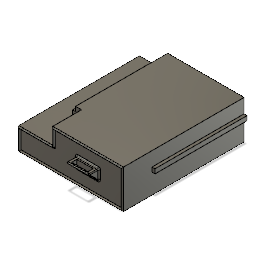
Drawer_for_ender3-pro_v14 (Autodesk Fusion 360 design; units mm, degrees)
Autodesk Fusion 360 part; units mm, degrees
sketch "Sketch1" plane through (0, 0, 0) normal (0, 0, 1) x (1, 0, 0)
  line L0 (0, 0) -> (-103, 0)
  line L1 (-103, 0) -> (-103, 52)
  line L2 (-103, 52) -> (0, 52)
  line L3 (0, 52) -> (0, 0)
  line L4 (0, 32.9) -> (4, 32.9)
  line L5 (4, 32.9) -> (4, 26.9)
  line L6 (4, 26.9) -> (0, 26.9)
  line L7 (-103, 46) -> (-107, 46)
  line L8 (-107, 46) -> (-107, 40)
  line L9 (-107, 40) -> (-103, 40)
  line L10 (-103, 30) -> (-141, 30)
  line L11 (-141, 30) -> (-141, 0)
  line L12 (-141, 0) -> (-103, 0)
  line L13 (-95, 52) -> (-95, 30)
  line L14 (-95, 30) -> (-103, 30)
  point P0 (0, 26.9)
  point P1 (0, 32.9)
  point P2 (-103, 40)
  point P3 (-103, 46)
  point P4 (-103, 30)
  point P5 (-95, 52)
  dimension "d1" = 103
  dimension "d2" = 52
  dimension "d3" = 26.9
  dimension "d4" = 6
  dimension "d5" = 4
  dimension "d6" = 40
  dimension "d7" = 6
  dimension "d8" = 4
  dimension "d9" = 30
  dimension "d10" = 38
  dimension "d11" = 8
  constraint horizontal L0
  constraint vertical L1
  constraint horizontal L2
  constraint vertical L3
  constraint coincident L0.start L3.end
  constraint coincident L3 P0
  constraint coincident L3 P1
  constraint coincident P1 L4.start
  constraint perpendicular L3 L4
  constraint perpendicular L4 L5
  constraint coincident P0 L6.end
  constraint perpendicular L3 L6
  constraint coincident L1 P2
  constraint coincident L1 P3
  constraint coincident P3 L7.start
  constraint horizontal L7
  constraint perpendicular L7 L8
  constraint coincident P2 L9.end
  constraint perpendicular L8 L9
  constraint coincident L1 P4
  constraint coincident P4 L10.start
  constraint perpendicular L1 L10
  constraint perpendicular L0 L11
  constraint perpendicular L1 L12
  constraint coincident L2 P5
  constraint coincident P5 L13.start
  constraint perpendicular L10 L13
  constraint perpendicular L1 L14
  measures "d1" distance of L0.start L0.end
  measures "d2" distance of L0.end L1.end
  measures "d3" distance of L0.start L6.end
  measures "d4" distance of P0 P1
  measures "d5" distance of P1 L4.end
  measures "d6" distance of L0.end L9.end
  measures "d7" distance of P2 P3
  measures "d8" distance of P3 L7.end
  measures "d9" distance of L0.end P4
  measures "d10" distance of P4 L10.end
  measures "d11" distance of L1.end P5
extrude "Extrude1" add sketch "Sketch1" along normal blind 164 contours L0 L1 L2 L3 L13 L14 | L1 L10 L11 L12 makes body 1
shell "Shell1" thickness 1.6 removed faces 1 at (-66, 10, 164) on bodies 1
extrude "Extrude2" add sketch "Sketch1" along normal blind 124 contours L3 L4 L5 L6 bodies 1
extrude "Extrude3" add sketch "Sketch1" along normal blind 124 contours L1 L2 L13 L14 | L1 L7 L8 L9 bodies 1
sketch "Sketch2" plane through (0, 0, 0) normal (0, 0, 1) x (1, 0, 0)
  line L0 (-95, 30) -> (-103, 30)
  line L1 (-95, 52) -> (-95, 30)
  line L2 (-95, 30) -> (-141, 30)
  line L3 (-141, 30) -> (-141, 0)
  line L4 (-141, 0) -> (0, 0)
  line L5 (0, 0) -> (0, 52)
  line L6 (0, 52) -> (-95, 52)
  line L7 (-93, 28) -> (-139, 28)
  line L8 (-139, 28) -> (-139, 2)
  line L9 (-139, 2) -> (-2, 2)
  line L10 (-2, 2) -> (-2, 50)
  line L11 (-2, 50) -> (-93, 50)
  line L12 (-93, 50) -> (-93, 28)
  point P0 (-95, 52)
  point P1 (-95, 30)
  point P2 (-141, 30)
  point P3 (-141, 0)
  point P4 (0, 52)
  dimension "d19" = 2
  constraint coincident P0 L1.start
  constraint coincident P1 L0.start
  constraint coincident P2 L2.end
  constraint coincident P3 L3.end
  constraint coincident L4.end L5.start
  constraint coincident P4 L5.end
extrude "Extrude4" add sketch "Sketch2" along normal blind 162.2 separate body contours L7 L8 L9 L10 L11 L12 makes body 2
shell "Shell2" thickness 1.6 removed faces 3 at (-32.3333, 50, 54.0667) at (-108.3333, 28, 108.1333) at (-93, 42.6667, 54.0667) on bodies 2
fillet "Fillet1" radius 1 10 edges at (-70.5, 2, 0) (-139, 15, 0) (-116, 28, 0) (-2, 26, 0) (-47.5, 50, 0) (-93, 39, 0) (-139, 28, 81.1) (-139, 2, 81.1) (-2, 2, 81.1) (-2, 50, 81.1) on bodies 2
fillet "Fillet2" radius 3 2 edges at (-93, 50, 1.3) (-92.7071, 49.7071, 0.2929) on bodies 2
fillet "Fillet3" radius 1 10 edges at (-115.5, 28, 162.2) (-138.7071, 27.7071, 162.2) (-139, 15, 162.2) (-138.7071, 2.2929, 162.2) (-70.5, 2, 162.2) (-2.2929, 2.2929, 162.2) (-2, 26, 162.2) (-2.2929, 49.7071, 162.2) (-48, 50, 162.2) (-93, 39, 162.2) on bodies 2
sketch "Sketch3" plane through (0, 0, 162.2) normal (0, 0, 1) x (1, 0, 0)
  line L0 (-3, 3) -> (-3, 49)
  line L1 (-3, 49) -> (-92, 49)
  line L2 (-92, 49) -> (-92, 27)
  line L3 (-92, 27) -> (-138, 27)
  line L4 (-138, 27) -> (-138, 3)
  line L5 (-138, 3) -> (-3, 3)
  line L6 (-33, 18.5) -> (-63, 18.5)
  line L7 (-63, 18.5) -> (-63, 33.5)
  line L8 (-63, 33.5) -> (-33, 33.5)
  line L9 (-33, 33.5) -> (-33, 18.5)
  line L10 (-33, 18.5) -> (-63, 33.5) construction
  line L11 (-63, 18.5) -> (-33, 33.5) construction
  point P0 (-48, 26)
  point P1 (-48, 26)
  point P2 (-48, 26)
  dimension "d34" = 30
  dimension "d35" = 15
  constraint coincident P2 P1
  constraint perpendicular L6 L7
  constraint parallel L6 L8
  constraint parallel L7 L9
  constraint horizontal L6
  constraint coincident L10 P2
  constraint coincident L11 P2
  measures "d34" distance of L7.end L8.end
  measures "d35" distance of L6.end L7.end
extrude "Extrude7" add sketch "Sketch3" along normal blind 15 contours L6 L7 L8 L9 bodies 2
sketch "Sketch5" plane through (-63, 0, 0) normal (-1, 0, 0) x (0, 0, 1)
  line L0 (162.2, 33.5) -> (162.2, 18.5)
  line L1 (162.2, 18.5) -> (177.2, 18.5)
  line L2 (177.2, 18.5) -> (177.2, 33.5)
  line L3 (177.2, 33.5) -> (162.2, 33.5)
  line L4 (162.2, 18.5) -> (177.2, 33.5)
  constraint coincident L0.end L1.start
  constraint coincident L2.end L3.start
extrude "Extrude8" cut sketch "Sketch5" against normal up to surface (30 mm away) contours L1 L2 L4 bodies 2
sketch "Sketch6" plane through (0, 33.5, 0) normal (0, 1, 0) x (-1, 0, 0)
  line L0 (33, 162.2) -> (63, 162.2)
  line L1 (63, 162.2) -> (63, 177.2)
  line L2 (63, 177.2) -> (33, 177.2)
  line L3 (33, 177.2) -> (33, 162.2)
  line L4 (59, 173.2) -> (37, 173.2)
  line L5 (37, 173.2) -> (37, 166.2)
  line L6 (37, 166.2) -> (59, 166.2)
  line L7 (59, 166.2) -> (59, 173.2)
  dimension "d40" = 4
extrude "Extrude9" cut sketch "Sketch6" against normal blind 20 contours L4 L5 L6 L7 bodies 2
fillet "Fillet6" radius 1 5 edges at (-63, 26, 169.7) (-48, 33.5, 177.2) (-33, 26, 169.7) (-33, 33.5, 169.7) (-63, 33.5, 169.7) on bodies 2
fillet "Fillet7" radius 2 8 edges at (-33.2929, 33.2071, 162.2) (-33, 26.2071, 162.2) (-33.2929, 18.9142, 162.2) (-48, 18.5, 162.2) (-62.7071, 18.9142, 162.2) (-63, 26.2071, 162.2) (-62.7071, 33.2071, 162.2) (-48, 33.5, 162.2) on bodies 2
sketch "Sketch7" plane through (0, 3.6, 0) normal (0, 1, 0) x (-1, 0, 0)
  line L0 (3.6, 1.6) -> (137.4, 1.6)
  line L1 (137.4, 1.6) -> (137.4, 160.6)
  line L2 (137.4, 160.6) -> (3.6, 160.6)
  line L3 (3.6, 160.6) -> (3.6, 1.6)
  line L4 (137.4, 93.6) -> (3.6, 93.6)
  line L5 (48.6, 1.6) -> (48.6, 93.6)
  line L6 (137.4, 41.6) -> (48.6, 41.6)
  line L7 (137.4, 95.2) -> (3.6, 95.2)
  line L8 (47, 1.6) -> (47, 93.6)
  line L9 (137.4, 43.2) -> (48.6, 43.2)
  dimension "d45" = 67
  dimension "d46" = 45
  dimension "d47" = 40
  dimension "d55" = 1.6
  dimension "d56" = 1.6
  dimension "d57" = 1.6
  constraint coincident L1 L4.start
  constraint coincident L3 L4.end
  constraint perpendicular L3 L4
  constraint coincident L0 L5.start
  constraint perpendicular L4 L5
  constraint coincident L1 L6.start
  constraint perpendicular L5 L6
  constraint coincident L5 L6.end
  constraint coincident L4 L5.end
  constraint coincident L1 L7.start
  constraint coincident L3 L7.end
  constraint perpendicular L3 L7
  constraint coincident L0 L8.start
  constraint coincident L4 L8.end
  constraint perpendicular L4 L8
  constraint coincident L1 L9.start
  constraint coincident L5 L9.end
  constraint perpendicular L5 L9
  measures "d45" distance of L1.end L4.start
  measures "d46" distance of L0.start L5.start
  measures "d47" distance of L0.end L6.start
  measures "d55" distance of L4.end L7.end
  measures "d56" distance of L5.start L8.start
  measures "d57" distance of L6.start L9.start
fillet "Fillet9" radius 1.5 6 edges at (-47.5, 52, 164) (-95, 41, 164) (-118, 30, 164) (-141, 15, 164) (-70.5, 0, 164) (0, 26, 164) on bodies 1
extrude "Extrude11" add sketch "Sketch7" along normal up to surface (24.4 mm away) contours L0 L4 L5 L8 | L1 L3 L4 L7 | L1 L5 L6 L9 bodies 2
named bodies: "outside", "inside"
